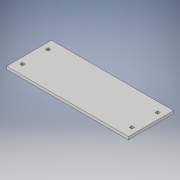
# Autodesk Inventor part: Part Atap
Saved by Autodesk Inventor 2019 (Build 230136000, 136)
## iProperties
Created: 2019-07-09
Part Number: Part Atap
Material: Generic
Document SubType Name: Modeling
Designer: azriel
Density: 1 g/cm^3
Appearance: Default
Author: azriel
Autodesk Inventor part; units mm, degrees
ref_plane "YZ Plane" through (0, 0, 0) normal (1, 0, 0) x (0, 1, 0)
ref_plane "XZ Plane" through (0, 0, 0) normal (0, 1, 0) x (-1, 0, 0)
ref_plane "XY Plane" through (0, 0, 0) normal (0, 0, 1) x (1, 0, 0)
sketch "Sketch1" plane through (0, 0, 0) normal (0, 1, 0) x (-1, 0, 0)
  line L0 (139.4119, -66.7225) -> (139.4119, -6.7225)
  line L1 (-80.5881, -6.7225) -> (-80.5881, -66.7225)
  line L2 (130.6619, -61.7225) -> (130.6619, -56.7225)
  line L3 (130.6619, -56.7225) -> (125.6619, -56.7225)
  line L4 (125.6619, -56.7225) -> (125.6619, -61.7225)
  line L5 (125.6619, -61.7225) -> (130.6619, -61.7225)
  line L6 (130.6619, -15.4975) -> (130.6619, -10.4975)
  line L7 (130.6619, -10.4975) -> (125.6619, -10.4975)
  line L8 (125.6619, -10.4975) -> (125.6619, -15.4975)
  line L9 (125.6619, -15.4975) -> (130.6619, -15.4975)
  line L10 (-71.8381, -61.7225) -> (-66.8381, -61.7225)
  line L11 (-66.8381, -61.7225) -> (-66.8381, -56.7225)
  line L12 (-66.8381, -56.7225) -> (-71.8381, -56.7225)
  line L13 (-71.8381, -56.7225) -> (-71.8381, -61.7225)
  line L14 (-71.8381, -15.4975) -> (-66.8381, -15.4975)
  line L15 (-66.8381, -15.4975) -> (-66.8381, -10.4975)
  line L16 (-66.8381, -10.4975) -> (-71.8381, -10.4975)
  line L17 (-71.8381, -10.4975) -> (-71.8381, -15.4975)
  line L18 (139.4119, -66.7225) -> (139.4119, -71.7225)
  line L19 (-80.5881, -71.7225) -> (-80.5881, -66.7225)
  line L20 (139.4119, -61.7225) -> (139.4119, -76.7225)
  line L21 (-80.5881, -76.7225) -> (-80.5881, -71.7225)
  line L22 (139.4119, -10.4975) -> (139.4119, 4.5025)
  line L23 (-80.5881, 4.5025) -> (-80.5881, -6.7225)
  line L24 (139.4119, -76.7225) -> (-80.5881, -76.7225)
  line L25 (139.4119, 4.5025) -> (-80.5881, 4.5025)
  point P0 (0, 0)
  dimension "d0" = 60
  dimension "d2" = 5
  dimension "d3" = 5
  dimension "d4" = 5
  dimension "d5" = 41.225
  dimension "d7" = 5
  dimension "d8" = 5
  dimension "d9" = 192.5
  dimension "d10" = 8.75
  dimension "d13" = 5
  constraints: 52 end point, 9 parallel, 5 perpendicular, 4 point on line, 4 vertical, 2 collinear, 1 horizontal
  measures "d0" distance of L0.start L0.end
  measures "d2" distance of L2.start L2.end
  measures "d3" distance of L3.end L2.end
  measures "d4" distance of L6.start L6.end
  measures "d5" distance between parallel lines of L9 L3
  measures "d7" distance of L10.start L10.end
  measures "d8" distance of L14.start L14.end
  measures "d9" distance between parallel lines of L11 L4
  measures "d10" distance between parallel lines of L1 L13
  measures "d13" distance of L0.start L18.end
extrude "Extrusion1" add sketch "Sketch1" along normal blind 5
body "Solid1"
